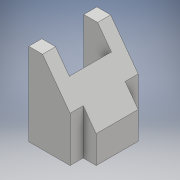
# Autodesk Inventor part: Part2
Saved by Autodesk Inventor 2018 (Build 220112000, 112)
## iProperties
Created: 2017-11-15
Part Number: Part2
Material: Generic
Document SubType Name: Modeling
Designer: kurti
Density: 1 g/cm^3
Appearance: Default
Author: kurti
Autodesk Inventor part; units mm, degrees
ref_plane "YZ Plane" through (0, 0, 0) normal (1, 0, 0) x (0, 1, 0)
ref_plane "XZ Plane" through (0, 0, 0) normal (0, 1, 0) x (-1, 0, 0)
ref_plane "XY Plane" through (0, 0, 0) normal (0, 0, 1) x (1, 0, 0)
sketch "Sketch1" plane through (0, 0, 0) normal (0, 0, 1) x (1, 0, 0)
  line L0 (-9.375, -11.75) -> (9.375, -11.75)
  line L1 (9.375, -11.75) -> (9.375, 11.75)
  line L2 (9.375, 11.75) -> (-9.375, 11.75)
  line L3 (-9.375, 11.75) -> (-9.375, -11.75)
  line L4 (-9.375, -11.75) -> (9.375, 11.75) construction
  line L5 (9.375, -11.75) -> (-9.375, 11.75) construction
  point P0 (0, 0)
  dimension "d0" = 18.75
  dimension "d1" = 23.5
  constraints: 12 end point, 2 midpoint, 2 parallel, 1 horizontal, 1 perpendicular
  measures "d0" distance of L1.end L2.end
  measures "d1" distance of L0.end L1.end
extrude "Extrusion1" add sketch "Sketch1" along normal blind 28.5
sketch "Sketch2" plane through (-9.375, 11.75, 0) normal (0, 1, 0) x (1, 0, 0)
  line L0 (0, -28.5) -> (18.75, -28.5) projected
  line L1 (0, -28.5) -> (4.75, -28.5)
  line L2 (18.75, 0) -> (18.75, -9.5)
  line L3 (18.75, 0) -> (18.75, -28.5) projected
  line L4 (18.75, -9.5) -> (4.75, -28.5)
  line L5 (18.75, -28.5) -> (4.75, -28.5)
  line L6 (18.75, -28.5) -> (18.75, -9.5)
  point P0 (9.375, 0)
  dimension "d4" = 4.75
  dimension "d5" = 9.5
  constraints: 10 end point, 2 point on line, 1 collinear, 1 perpendicular
  measures "d4" distance of L0.start L1.end
  measures "d5" distance of L2.start L2.end
extrude "Extrusion2" cut sketch "Sketch2" against normal blind 28.5
sketch "Sketch7" plane through (-9.375, 11.75, 0) normal (0, 1, 0) x (1, 0, 0)
  line L0 (18.75, 0) -> (18.75, -9.5) projected
  line L1 (18.75, -9.5) -> (18.75, 0)
  line L2 (18.75, 0) -> (14.25, 0)
  line L3 (0, 0) -> (18.75, 0) projected
  line L4 (14.25, 0) -> (14.25, -15.6071)
  line L5 (18.75, -9.5) -> (4.75, -28.5) projected
  line L6 (18.75, -9.5) -> (14.25, -15.6071)
  point P0 (9.375, 0)
  dimension "d27" = 4.5
  constraints: 8 end point, 2 collinear, 1 point on line, 1 vertical
  measures "d27" distance of L0.start L2.end
extrude "Extrusion7" cut sketch "Sketch7" against normal blind 4.5
sketch "Sketch8" plane through (-9.375, -11.75, 0) normal (0, -1, 0) x (1, 0, 0)
  line L0 (18.75, 0) -> (18.75, 9.5) projected
  line L1 (18.75, 0) -> (14.25, 0)
  line L2 (0, 0) -> (18.75, 0) projected
  line L3 (18.75, 9.5) -> (14.25, 15.6071) projected
  line L4 (14.25, 0) -> (14.25, 15.6071)
  line L5 (14.25, 15.6071) -> (18.75, 9.5)
  line L6 (18.75, 0) -> (18.75, 9.5)
  point P0 (9.375, 0)
  dimension "d30" = 4.5
  constraints: 8 end point, 2 point on line, 1 parallel
  measures "d30" distance of L0.start L1.end
extrude "Extrusion8" cut sketch "Sketch8" against normal blind 4.5
sketch "Sketch9" plane through (-9.375, -11.75, 0) normal (-1, 0, 0) x (0, 0, 1)
  line L0 (15.6071, 19) -> (0, 19) projected
  line L1 (28.5, 4.5) -> (0, 4.5)
  line L2 (0, 4.5) -> (0, 19)
  line L3 (0, 19) -> (28.5, 19)
  line L4 (28.5, 19) -> (28.5, 4.5)
  line L5 (28.5, 23.5) -> (28.5, 0) projected
  line L6 (0, 0) -> (28.5, 0) projected
  point P0 (0, 11.75)
  dimension "d35" = 0
  dimension "d36" = 4.5
  constraints: 8 end point, 2 parallel, 1 horizontal, 1 perpendicular
  measures "d35" distance between parallel lines of L5 L4
  measures "d36" distance between parallel lines of L6 L1
extrude "Extrusion9" cut sketch "Sketch9" against normal blind 9.5
body "Solid1"
